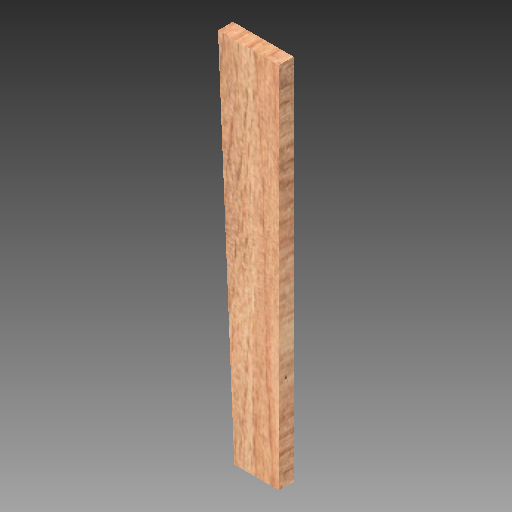
# Autodesk Inventor part: internalSupportTop4
Saved by Autodesk Inventor 2019 (Build 230136000, 136)
## iProperties
Company: FABLAB Torino
Created: 2019-01-11
Part Number: internalSupportTop4
Material: Wood (Birch)
Document SubType Name: Modeling
Designer: Giancarlo
Density: 0.55 g/cm^3
Appearance: Birch - Natural Polished
Description: MultiLayer 10mm
Author: Giancarlo
Title: La Panca - Flower Vase
Subject: Construction MOld
Autodesk Inventor part; units mm, degrees
ref_plane "YZ Plane" through (0, 0, 0) normal (1, 0, 0) x (0, 1, 0)
ref_plane "XZ Plane" through (0, 0, 0) normal (0, 1, 0) x (-1, 0, 0)
ref_plane "Work Plane1" through (0, 0, 0) normal (0, 0, 1) x (1, 0, 0)
sketch "Sketch1" plane through (0, 0, 0) normal (0, 0, 1) x (1, 0, 0)
  line L0 (0, 3) -> (29.1929, 3) construction
  line L1 (29.1929, 3) -> (80.018, 3) construction
  line L2 (80.018, 3) -> (80.018, 0) construction
  line L3 (80.018, 0) -> (29.1929, 0) construction
  line L4 (29.1929, 0) -> (29.1929, 3) construction
  line L5 (0, 0) -> (0, 3) construction
  line L6 (29.1929, 0) -> (0, 0) construction
  spline S0 degree 3 poles (-12.886, 247) (-12.5523, 247.0134) (-12.2186, 247.0269) (-11.5512, 247.0537) (-11.2175, 247.0672) (-10.8837, 247.0806) knots -0.200389 -0.200389 -0.200389 -0.200389 -0.100195 -0.100195 0 0 0 0 construction
  spline S1 degree 3 poles (-0.9779, -0.0396) (-1.3117, -0.0528) (-1.6454, -0.0659) (-2.3129, -0.0923) (-2.6467, -0.1055) (-2.9805, -0.1187) knots -0.200408 -0.200408 -0.200408 -0.200408 -0.100204 -0.100204 0 0 0 0 construction
  line L7 (29.1929, 0) -> (-0.9779, -0.0396)
  line L8 (28.8688, 247.1327) -> (29.1929, 0)
  line L9 (117.4636, 247.2359) -> (117.4688, 243.2359) construction
  line L10 (117.4688, 243.2359) -> (95.3505, 243.2069) construction
  line L11 (95.3505, 243.2069) -> (95.3452, 247.2069) construction
  line L12 (95.3452, 247.2069) -> (117.4636, 247.2359) construction
  spline S2 degree 3 poles (-11.8803, 243.0663) (-11.8811, 243.7329) (-11.882, 244.3996) (-11.8838, 245.7329) (-11.8846, 246.3996) (-11.8855, 247.0663) knots -0.4 -0.4 -0.4 -0.4 -0.2 -0.2 0 0 0 0 construction
  line L13 (-11.8855, 247.0663) -> (85.2837, 247.1937) construction
  line L14 (85.2837, 247.1937) -> (85.2889, 243.1937) construction
  line L15 (85.2889, 243.1937) -> (-11.8803, 243.0663) construction
  line L16 (28.8688, 247.1327) -> (-11.8855, 247.0663)
  line L17 (-11.8855, 247.0663) -> (-0.9779, -0.0396)
  constraints: 36 end point, 4 horizontal, 3 vertical, 1 perpendicular, 33 other
extrude "Extrusion1" add sketch "Sketch1" along normal blind 10
body "Solid1"
